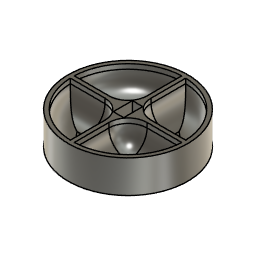
V1 dispensador v1 (Autodesk Fusion 360 design; units mm, degrees)
Autodesk Fusion 360 part; units mm, degrees
sketch "Sketch1" plane through (0, 0, 0) normal (0, 0, 1) x (1, 0, 0)
  circle A0 centre (0, 0) radius 75
  line L0 (0, 0) -> (75, 0)
  line L1 (75, 0) -> (75, 3)
  line L2 (75, 3) -> (75, -3)
  line L3 (-75, 0) -> (-75, 2.5)
  line L4 (-75, 2.5) -> (-75, -2.5)
  line L5 (-75, -2.5) -> (80, -2.5)
  line L6 (80, -2.5) -> (80, 2.5)
  line L7 (80, 2.5) -> (-75, 2.5)
  dimension "d1" = 150
  dimension "d2" = 3
  dimension "d3" = 6
  dimension "d4" = 2.5
  dimension "d5" = 5
  dimension "d6" = 5
  constraint coincident A0.centre L0.start
  constraint coincident A0 L0.end
  constraint horizontal L0
  constraint perpendicular L0 L1
  constraint perpendicular L0 L2
  constraint coincident A0 L3.start
  constraint vertical L3
  constraint parallel L3 L4
  constraint perpendicular L4 L5
  constraint perpendicular L5 L6
  measures "d1" diameter of A0
  measures "d2" distance of L0.end L1.end
  measures "d3" distance of L1.end L2.end
  measures "d4" distance of L3.start L3.end
  measures "d5" distance of L3.end L4.end
  measures "d6" distance of L5.end L6.end
extrude "Extrude1" add sketch "Sketch1" along normal blind 5 contours A0 L5 L7 | A0 L7 | A0 L5 makes body 1
sketch "Sketch2" plane through (0, 0, 5) normal (0, 0, 1) x (-1, 0, 0)
  circle A0 centre (0, 0) radius 75
  line L0 (0, 0) -> (-75, 0)
  line L1 (-75, 0) -> (-75, -2.5)
  line L2 (-75, -2.5) -> (-75, 2.5)
  line L3 (-75, 2.5) -> (78.1024, 2.5)
  line L4 (78.1024, 2.5) -> (78.1024, -2.5)
  line L5 (78.1024, -2.5) -> (-75, -2.5)
  line L6 (0, -75) -> (-2.5, -75)
  line L7 (-2.5, -75) -> (2.5, -75)
  line L8 (2.5, -75) -> (2.5, 77.5039)
  line L9 (2.5, 77.5039) -> (-2.5, 77.5039)
  line L10 (-2.5, 77.5039) -> (-2.5, -75)
  circle A1 centre (0, 0) radius 70
  dimension "d9" = 90
  dimension "d10" = 2.5
  dimension "d11" = 5
  dimension "d12" = 5
  dimension "d13" = 2.5
  dimension "d14" = 5
  dimension "d15" = 5
  constraint coincident A0.centre L0.start
  constraint coincident A0 L0.end
  constraint horizontal L0
  constraint perpendicular L0 L2
  constraint perpendicular L2 L3
  constraint perpendicular L3 L4
  constraint coincident A0 L6.start
  constraint parallel L0 L6
  constraint parallel L6 L7
  constraint vertical L8
  constraint perpendicular L8 L9
  measures "d9" angle of L0 L1
  measures "d10" distance of L0.end L1.end
  measures "d11" distance of L1.end L2.end
  measures "d12" distance of L3.end L4.end
  measures "d13" distance of L6.start L6.end
  measures "d14" distance of L6.end L7.end
  measures "d15" distance of L8.end L9.end
extrude "Extrude2" add sketch "Sketch2" along normal blind 30 separate body contours A0 L3 L5 A1 | A0 L3 L8 A1 | A0 L5 L8 A1 | L3 L5 L8 A1 | A0 L8 L10 A1 | A0 L3 L10 A1 | L3 L8 L10 A1 | L3 L5 L8 L10 | L5 L8 L10 A1 | A0 L0 L3 A1 | L0 L3 L10 A1 | A0 L5 L10 A1 | L0 L5 L10 A1 | A0 L0 L5 A1 picked at (0, -71.6634) makes body 2
extrude "Extrude3" add sketch "Sketch2" along normal blind 30 contours A0 L8 L10 A1 picked at (-1.9445, 71.6362) bodies 1 2
fillet "Fillet1" radius 24 4 edges at (-2.5, 36.2277, 5) (-2.5, 2.5, 20) (-36.2277, 2.5, 5) (-49.4975, 49.4975, 5) on bodies 1
fillet "Fillet2" radius 24 10 edges at (-36.2277, -2.5, 5) (-2.5, -2.5, 20) (-2.5, -36.2277, 5) (-49.4975, -49.4975, 5) (49.4975, -49.4975, 5) (2.5, -36.2277, 5) (36.2277, 2.5, 5) (2.5, 36.2277, 5) (36.2277, -2.5, 5) (49.4975, 49.4975, 5) on bodies 1
fillet "Fillet3" radius 24 4 edges at (9.5294, -9.5294, 12.0294) (2.5, -2.5, 32) (9.5294, 9.5294, 12.0294) (2.5, 2.5, 32) on bodies 1
sketch "Sketch3" plane through (0, 0, 0) normal (0, 0, -1) x (1, 0, 0)
  circle A0 centre (0, 0) radius 75
  line L0 (-34.5, -27) -> (34.5, -27)
  line L1 (34.5, -27) -> (34.5, 27)
  line L2 (34.5, 27) -> (-34.5, 27)
  line L3 (-34.5, 27) -> (-34.5, -27)
  line L4 (-34.5, -27) -> (34.5, 27) construction
  line L5 (34.5, -27) -> (-34.5, 27) construction
  dimension "d26" = 69
  dimension "d27" = 54
  constraint horizontal L0
  constraint perpendicular L0 L1
  constraint parallel L0 L2
  constraint parallel L1 L3
  constraint coincident L4 A0.centre
  constraint coincident L5 A0.centre
  constraint coincident A0.centre origin
  measures "d26" distance of L1.end L2.end
  measures "d27" distance of L0.end L1.end
extrude "Extrude4" cut sketch "Sketch3" against normal blind 4 contours L0 L1 L2 L3 bodies 1
extrude "Extrude5" add 1 faces at (1.8683, 42.9301, 0) along direction (0, 0, -1) blind 6 on bodies 1 bodies 1
sketch "Sketch4" plane through (0, 0, 35) normal (0, 0, 1) x (-1, 0, 0)
  circle A0 centre (0, 0) radius 75
  line L0 (-2.5, 69.9553) -> (-2.5, 26.5)
  arc A1 (-26.5, 2.5) -> (-2.5, 26.5) centre (-26.5, 26.5) ccw
  line L1 (-26.5, 2.5) -> (-69.9553, 2.5)
  arc A2 (-2.5, 69.9553) -> (-69.9553, 2.5) centre (0, 0) ccw
  line L2 (-69.9553, -2.5) -> (-26.5, -2.5)
  arc A3 (-2.5, -26.5) -> (-26.5, -2.5) centre (-26.5, -26.5) ccw
  line L3 (-2.5, -26.5) -> (-2.5, -69.9553)
  arc A4 (-69.9553, -2.5) -> (-2.5, -69.9553) centre (0, 0) ccw
  line L4 (26.5, -2.5) -> (69.9553, -2.5)
  arc A5 (2.5, -69.9553) -> (69.9553, -2.5) centre (0, 0) ccw
  line L5 (2.5, -69.9553) -> (2.5, -26.5)
  arc A6 (26.5, -2.5) -> (2.5, -26.5) centre (26.5, -26.5) ccw
  arc A7 (69.9553, 2.5) -> (2.5, 69.9553) centre (0, 0) ccw
  line L6 (69.9553, 2.5) -> (26.5, 2.5)
  arc A8 (2.5, 26.5) -> (26.5, 2.5) centre (26.5, 26.5) ccw
  line L7 (2.5, 26.5) -> (2.5, 69.9553)
  line L8 (-6.5, -12) -> (6.5, -12)
  line L9 (6.5, -12) -> (6.5, 12)
  line L10 (6.5, 12) -> (-6.5, 12)
  line L11 (-6.5, 12) -> (-6.5, -12)
  line L12 (-6.5, -12) -> (6.5, 12) construction
  line L13 (6.5, -12) -> (-6.5, 12) construction
  dimension "d32" = 13
  dimension "d33" = 24
  constraint horizontal L8
  constraint perpendicular L8 L9
  constraint parallel L8 L10
  constraint parallel L9 L11
  constraint coincident L12 A0.centre
  constraint coincident L13 A0.centre
  constraint coincident A0.centre A2.centre
  measures "d32" distance of L9.end L10.end
  measures "d33" distance of L8.end L9.end
extrude "Extrude6" cut sketch "Sketch4" against normal blind 29 contours L8 L9 L10 L11 bodies 1
sketch "Sketch5" plane through (0, 0, 4) normal (0, 0, -1) x (1, 0, 0)
  line L0 (-34.5, 27) -> (-34.5, -27)
  line L1 (-34.5, -27) -> (34.5, -27)
  line L2 (34.5, -27) -> (34.5, 27)
  line L3 (34.5, 27) -> (-34.5, 27)
  circle A0 centre (0, 0) radius 4
  constraint coincident A0.centre origin
extrude "Extrude7" cut sketch "Sketch5" against normal blind 1000 contours A0 bodies 1
sketch "Sketch6" plane through (0, 0, -6) normal (0, 0, -1) x (1, 0, 0)
  line L0 (34.5, -27) -> (-34.5, -27)
  line L1 (-34.5, -27) -> (-34.5, 27)
  line L2 (-34.5, 27) -> (34.5, 27)
  line L3 (34.5, 27) -> (34.5, -27)
  circle A0 centre (0, 0) radius 75
  line L4 (-34.5, 0) -> (-34.5, -10)
  line L5 (-34.5, -10) -> (-83.4898, -10)
  line L6 (-83.4898, -10) -> (-83.4898, 10)
  line L7 (-83.4898, 10) -> (-34.5, 10)
  line L8 (-34.5, 10) -> (-34.5, -10)
  dimension "d38" = 20
  constraint midpoint L1 L4.start
  constraint coincident L1 L4.end
  constraint parallel L1 L4
  constraint horizontal L5
  constraint vertical L6
  constraint horizontal L7
  constraint vertical L8
  measures "d38" distance of L4.end L7.end
extrude "Extrude8" cut sketch "Sketch6" against normal blind 10 contours L1 A0 L4 L5 L7 L8 bodies 1
